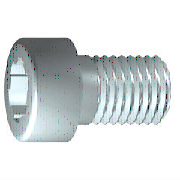
# Autodesk Inventor part: ANSI B18.3 - 4-40 UNC - 0.25, SSHCSI
Saved by Autodesk Inventor 2023.2 (Build 272271000, 271)
## iProperties
Created: 2022-02-04
Part Number: ANSI B18.3 - 4-40 UNC - 0.25, SSHCSI
Material: Steel, Mild
Description: Hexagon Socket Head Cap Screw
Document SubType Name: Modeling
Standard: ANSI B18.3
Designer: Nathan Cai
Standard Revision: 2003
Standards Organization: ANSI
Language: en-US
Size Designation: 4-40 UNC - 0.25
Categories: <MemberInstance><Categories><Category DisplayName="Fasteners" InternalName="e4da775c-781d-43d5-af7c-5136215cf5a6" Mnemonic="FSTN"><Category DisplayName="Bolts" InternalName="536e6df0-f778-49ac-b2f2-25c71d2aa0b2" Mnemonic="SCRW"><CategoryParameter DisplayName="Nominal Diameter Designation" InternalName="03caf894-eafd-4c09-a035-916ac084b87b" Mnemonic="nomdiadesig"/><CategoryParameter DisplayName="Nominal Length" InternalName="238ecbaf-3e6c-45dd-aa95-4068c8e0fd02" Mnemonic="nomlen"/><CategoryParameter DisplayName="Thread Designation" InternalName="586d5e89-370a-4089-914f-0110033585c7" Mnemonic="thrdesign"/><CategoryParameter DisplayName="Thread Series Designation" InternalName="87c5849c-b3a5-4c3e-9c9b-2feecef9be86" Mnemonic="thrserdsgn"/><CategoryParameter DisplayName="Nominal Diameter" InternalName="8bbe3f8e-44cf-40a9-a251-3a6edc8168d6" Mnemonic="nomdia"/><CategoryParameter DisplayName="Thread Type" InternalName="b4bbb7bc-d6aa-4c9f-a9a9-4152b9f6fe49" Mnemonic="thrtype"/><CategoryParameter DisplayName="Thread Pitch" InternalName="bb82302e-82d8-4176-8fc1-c5d7bb17d5ad" Mnemonic="pitch1"/><CategoryParameter DisplayName="Threads per Unit" InternalName="bdc6e7d2-ffd0-4d9c-a173-16b95ebb912d" Mnemonic="thrperunit1"/><CategoryParameter DisplayName="Thread Class" InternalName="ebc0d23b-2cc6-4d2a-b376-d52aae53bab6" Mnemonic="thrclss"/><Category DisplayName="Socket Head" InternalName="55e06bf3-7e58-486c-bbdc-745fcc60664d" Mnemonic="CLSCRW"><CategoryParameter DisplayName="Shank Diameter" InternalName="179dbae3-102f-48bb-85fe-1e3ecd34f7cc" Mnemonic="grpdia"/><CategoryParameter DisplayName="Thread Length" InternalName="3268731d-5f9a-4750-8b01-4a959c46fbf2" Mnemonic="thrlen"/><CategoryParameter DisplayName="Head Diameter" InternalName="46177176-dbdd-4a1b-aefd-4c60c45016af" Mnemonic="headdia"/><CategoryParameter DisplayName="Grip Length" InternalName="52eab69f-422f-4795-9995-175a1b827e67" Mnemonic="grplen"/><CategoryParameter DisplayName="Type" InternalName="59a7e495-7a0c-4a5c-bdfd-c090c5f6e2db" Mnemonic="type"/><CategoryParameter DisplayName="Head Height" InternalName="99c92c4c-4a02-4ebe-9e64-948fb169e19e" Mnemonic="headh"/></Category></Category></Category><Category DisplayName="DataType" InternalName="23b78d0f-2648-40c6-8793-ca6db495c9e8" Mnemonic="DATATYPE"><CategoryParameter DisplayName="DisplayName" InternalName="05415f3d-3907-474b-a020-eb9d644f4cf3" Mnemonic="DISPLAYNAME"/><CategoryParameter DisplayName="Standard" InternalName="0c0a119c-1e12-4c84-803f-101930972f5e" Mnemonic="STANDARD"/><CategoryParameter DisplayName="Description" InternalName="13903e3d-64b1-4950-80da-f627842ea37f" Mnemonic="DESCRIPTION"/><CategoryParameter DisplayName="Designation" InternalName="2675968c-4ce5-49e0-a4f5-552d29089031" Mnemonic="DESIGNATION"/><CategoryParameter DisplayName="Default Row" InternalName="2af9ec52-faaa-4026-b378-f9fa4afca842" Mnemonic="DEFAULTROW"/><CategoryParameter DisplayName="Folder Name" InternalName="3f06958e-8713-4116-9be7-ed6184ecc97b" Mnemonic="FOLDERNAME"/><CategoryParameter DisplayName="Revision Guid" InternalName="45a75005-10b1-4dfc-8d6d-dfe629f0b93c" Mnemonic="REVISIONGUID"/><CategoryParameter DisplayName="FileName" InternalName="8b46a4cc-9585-4fed-90c3-899f57e09a73" Mnemonic="FILENAME"/><CategoryParameter DisplayName="StdsOrg" InternalName="8f5914e1-4693-403f-8ab5-d37768198c9d" Mnemonic="STDSORG"/><CategoryParameter DisplayName="Family Version" InternalName="914462f6-6e19-4b14-ba84-155b9680b1d0" Mnemonic="FAMILYREVISION"/><CategoryParameter DisplayName="Standard Revision" InternalName="91d5a463-65c2-4fde-b823-3b7fea5e8e17" Mnemonic="STANDARDREVISION"/><CategoryParameter DisplayName="Member Revision" InternalName="a65d44b9-392f-4f4f-857b-e4b3d54996fe" Mnemonic="MEMBERREVISION"/><CategoryParameter DisplayName="ClipFormat" InternalName="bc51e27b-3422-4e78-93ef-cec197ddf230" Mnemonic="CLIPFORMAT"/><CategoryParameter DisplayName="Manufacturer" InternalName="cd6c7a72-a28a-4e50-99a9-2c7f4e13e5ad" Mnemonic="MANUFACTURER"/><CategoryParameter DisplayName="InternalName" InternalName="cf1d0246-76d9-4b4a-8305-fa0409afb5c1" Mnemonic="INTERNALNAME"/><CategoryParameter DisplayName="IsMetric" InternalName="e2385c5b-1ea4-4823-96a8-8de651266ec3" Mnemonic="ISMETRIC"/><Category DisplayName="Part" InternalName="c0e0b642-3bcb-4cc8-9e80-f96d35c4afa4" Mnemonic="PART"><CategoryParameter DisplayName="Part Number" InternalName="016b6077-bfbe-49bd-92c9-d8d59c39c941" Mnemonic="PARTNUMBER"/><CategoryParameter DisplayName="Stock Number" InternalName="4dba7c1c-e26c-444e-836c-b08b433409a8" Mnemonic="STOCKNUMBER"/><CategoryParameter DisplayName="Material Key" InternalName="5c9a8adb-dd2b-4535-b97f-0a94a95fe41f" Mnemonic="MATERIALKEY"/><CategoryParameter DisplayName="Material" InternalName="818a152a-d3c3-49ca-80ee-df7d91421b8e" Mnemonic="MATERIAL"/></Category></Category><Category DisplayName="Legacy Map DA" InternalName="924fff40-ddd0-4eff-ad42-30e3774ef79e" Mnemonic="LEGACYMAPDA"><CategoryParameter DisplayName="DACookie" InternalName="316934ee-8fe1-4c7a-9c36-f2d79e1add1a" Mnemonic="DACOOKIE"/></Category><Category DisplayName="LegacyMap" InternalName="cd87c42b-3e48-431e-b5c0-1cbeb14dfe77" Mnemonic="LEGACYMAP"><CategoryParameter DisplayName="unique DA member ID" InternalName="0918ad47-427f-4fed-ae26-24c81c58f590" Mnemonic="DACOOKIE"/><CategoryParameter DisplayName="Merge11 ID" InternalName="0ee8fb18-e2ed-4f39-96f6-1f4b5f50aa71" Mnemonic="MERGE11"/><CategoryParameter DisplayName="unique CC member ID" InternalName="5193edd4-b2b0-4ab4-9d54-de900eee34e0" Mnemonic="CCCOOKIE"/><CategoryParameter DisplayName="Split ID" InternalName="72b5c83c-be7f-45c4-ae51-9160ea6deb26" Mnemonic="SPLIT"/><CategoryParameter DisplayName="MemberID" InternalName="8e5e0294-fc51-4c8f-b3d7-003dc5ed94f6" Mnemonic="MEMBERID"/><CategoryParameter DisplayName="CatalogName" InternalName="d99d1e27-aa94-4de2-af4c-c348882a6f4f" Mnemonic="CATALOGNAME"/><CategoryParameter DisplayName="FamilyNumber" InternalName="e705e1f4-09cb-413e-91f9-551b4188271e" Mnemonic="FAMILYNUMBER"/></Category></Categories><FamilyTemplate Id="sis145"><FamilyTemplateParameters><FamilyTemplateParameter ObjectType="kUserParameterObject" ValueType="xs:double" Id="1" ObjectReferenceKey="GUL"/><FamilyTemplateParameter ObjectType="kUserParameterObject" ValueType="xs:double" Id="2" ObjectReferenceKey="KOH"/><FamilyTemplateParameter ObjectType="kUserParameterObject" ValueType="xs:double" Id="3" ObjectReferenceKey="NLG"/><FamilyTemplateParameter ObjectType="kUserParameterObject" ValueType="xs:double" Id="4" ObjectReferenceKey="KOD"/><FamilyTemplateParameter ObjectType="kUserParameterObject" ValueType="xs:double" Id="5" ObjectReferenceKey="SBR"/><FamilyTemplateParameter ObjectType="kUserParameterObject" ValueType="xs:double" Id="6" ObjectReferenceKey="TOA"/><FamilyTemplateParameter ObjectType="kUserParameterObject" ValueType="xs:double" Id="7" ObjectReferenceKey="GD1"/><FamilyTemplateParameter ObjectType="kUserParameterObject" ValueType="xs:double" Id="8" ObjectReferenceKey="GEL"/><FamilyTemplateParameter ObjectType="kUserParameterObject" ValueType="xs:double" Id="9" ObjectReferenceKey="SW"/><FamilyTemplateParameter ObjectType="kUserParameterObject" ValueType="xs:double" Id="10" ObjectReferenceKey="THREADDIA"/><FamilyTemplateParameter ObjectType="kUserParameterObject" ValueType="xs:double" Id="11" ObjectReferenceKey="SPD"/><FamilyTemplateParameter ObjectType="kUserParameterObject" ValueType="xs:double" Id="12" ObjectReferenceKey="INTI"/><FamilyTemplateParameter ObjectType="kUserParameterObject" ValueType="xs:double" Id="13" ObjectReferenceKey="BDM"/><FamilyTemplateParameter ObjectType="kUserParameterObject" ValueType="xs:double" Id="14" ObjectReferenceKey="ANZ"/><FamilyTemplateParameter ObjectType="kUserParameterObject" ValueType="xs:double" Id="15" ObjectReferenceKey="RR"/><FamilyTemplateParameter ObjectType="kUserParameterObject" ValueType="xs:double" Id="16" ObjectReferenceKey="TPU"/><FamilyTemplateParameter ObjectType="kUserParameterObject" ValueType="xs:double" Id="17" ObjectReferenceKey="PTC"/><FamilyTemplateParameter ObjectType="kUserParameterObject" ValueType="xs:double" Id="18" ObjectReferenceKey="NND"/><FamilyTemplateParameter ObjectType="kUserParameterObject" ValueType="xs:double" Id="19" ObjectReferenceKey="GD"/><FamilyTemplateParameter ObjectType="kUserParameterObject" ValueType="xs:double" Id="20" ObjectReferenceKey="GAL"/><FamilyTemplateParameter ObjectType="kUserParameterObject" ValueType="xs:double" Id="21" ObjectReferenceKey="E0"/><FamilyTemplateParameter ObjectType="kPropertyObject" ValueType="xs:string" Id="100" ObjectReferenceKey="{32853F0F-3444-11d1-9E93-0060B03C1CA6}" SubObjectId="52"/><FamilyTemplateParameter ObjectType="kPropertyObject" ValueType="xs:string" Id="105" ObjectReferenceKey="{32853F0F-3444-11d1-9E93-0060B03C1CA6}" SubObjectId="5"/><FamilyTemplateParameter ObjectType="kPartComponentDefinitionObject" ValueType="xs:string" Id="110" SubObjectId="Material"/><FamilyTemplateParameter ObjectType="kThreadFeatureObject" ValueType="xs:structure" Id="300" ObjectReferenceKey="100200001000000000100000000000008000000000000000" SubObjectId="ThreadInfo"><FamilyTemplateParameter ObjectType="" ValueType="xs:string" Id="301" SubObjectId="ThreadDesignation"/><FamilyTemplateParameter ObjectType="" ValueType="xs:string" Id="302" SubObjectId="ThreadType"/><FamilyTemplateParameter ObjectType="" ValueType="xs:string" Id="303" SubObjectId="ThreadClass"/></FamilyTemplateParameter></FamilyTemplateParameters></FamilyTemplate><CategoryParameterMap><ParamToTemplateMap><ParamToTemplate CategoryParameter="//CategoryParameter[@InternalName='05415f3d-3907-474b-a020-eb9d644f4cf3']" ConstantValue="Spline Socket Head Cap Screw - Inch"/><ParamToTemplate CategoryParameter="//CategoryParameter[@InternalName='cf1d0246-76d9-4b4a-8305-fa0409afb5c1']" ConstantValue="48533e16-23c5-4596-a6af-3b71bb979595"/><ParamToTemplate CategoryParameter="//CategoryParameter[@InternalName='3f06958e-8713-4116-9be7-ed6184ecc97b']" ConstantValue="ANSI B18.3(13)"/><ParamToTemplate CategoryParameter="//CategoryParameter[@InternalName='914462f6-6e19-4b14-ba84-155b9680b1d0']" ConstantValue="10"/><ParamToTemplate CategoryParameter="//CategoryParameter[@InternalName='bc51e27b-3422-4e78-93ef-cec197ddf230']" ConstantValue="CF_INVENTOR.STDPARTS"/><ParamToTemplate CategoryParameter="//CategoryParameter[@InternalName='e2385c5b-1ea4-4823-96a8-8de651266ec3']" ConstantValue="false"/><ParamToTemplate CategoryParameter="//CategoryParameter[@InternalName='13903e3d-64b1-4950-80da-f627842ea37f']" ConstantValue="Hexagon Socket Head Cap Screw"/><ParamToTemplate CategoryParameter="//CategoryParameter[@InternalName='8f5914e1-4693-403f-8ab5-d37768198c9d']" ConstantValue="ANSI"/><ParamToTemplate CategoryParameter="//CategoryParameter[@InternalName='0c0a119c-1e12-4c84-803f-101930972f5e']" ConstantValue="ANSI B18.3"/><ParamToTemplate CategoryParameter="//CategoryParameter[@InternalName='cd6c7a72-a28a-4e50-99a9-2c7f4e13e5ad']" TemplateParameter="104"/><ParamToTemplate CategoryParameter="//CategoryParameter[@InternalName='91d5a463-65c2-4fde-b823-3b7fea5e8e17']" ConstantValue="2003"/><ParamToTemplate CategoryParameter="//CategoryParameter[@InternalName='45a75005-10b1-4dfc-8d6d-dfe629f0b93c']" ConstantValue="427e49c2-ecb5-4fa3-b939-1b6f11ba86db"/><ParamToTemplate CategoryParameter="//CategoryParameter[@InternalName='2af9ec52-faaa-4026-b378-f9fa4afca842']" ConstantValue="110"/><ParamToTemplate CategoryParameter="//CategoryParameter[@InternalName='d99d1e27-aa94-4de2-af4c-c348882a6f4f']" ConstantValue="ANSI"/><ParamToTemplate CategoryParameter="//CategoryParameter[@InternalName='8b46a4cc-9585-4fed-90c3-899f57e09a73']" ConstantValue="ANSI B18.3 - 4-40 UNC - 0.25(22)"/><ParamToTemplate CategoryParameter="//CategoryParameter[@InternalName='a65d44b9-392f-4f4f-857b-e4b3d54996fe']" ConstantValue="0708E7DF-237C-4B0D-ACF9-FA1811921CFF"/><ParamToTemplate CategoryParameter="//CategoryParameter[@InternalName='52eab69f-422f-4795-9995-175a1b827e67']" ConstantValue="0.0625"/><ParamToTemplate CategoryParameter="//CategoryParameter[@InternalName='ebc0d23b-2cc6-4d2a-b376-d52aae53bab6']" ConstantValue="2A"/><ParamToTemplate CategoryParameter="//CategoryParameter[@InternalName='87c5849c-b3a5-4c3e-9c9b-2feecef9be86']" ConstantValue="UNC"/><ParamToTemplate CategoryParameter="//CategoryParameter[@InternalName='03caf894-eafd-4c09-a035-916ac084b87b']" ConstantValue="#4"/><ParamToTemplate CategoryParameter="//CategoryParameter[@InternalName='b4bbb7bc-d6aa-4c9f-a9a9-4152b9f6fe49']" ConstantValue="ANSI Unified Screw Threads"/><ParamToTemplate CategoryParameter="//CategoryParameter[@InternalName='e705e1f4-09cb-413e-91f9-551b4188271e']" ConstantValue="155"/><ParamToTemplate CategoryParameter="//CategoryParameter[@InternalName='8e5e0294-fc51-4c8f-b3d7-003dc5ed94f6']" ConstantValue="4040"/><ParamToTemplate CategoryParameter="//CategoryParameter[@InternalName='316934ee-8fe1-4c7a-9c36-f2d79e1add1a']" ConstantValue="*Ans~AB18_3_2~No. 4-40x0.25~0.25~UNRC*"/><ParamToTemplate CategoryParameter="//CategoryParameter[@InternalName='179dbae3-102f-48bb-85fe-1e3ecd34f7cc']" TemplateParameter="13"/><ParamToTemplate CategoryParameter="//CategoryParameter[@InternalName='2675968c-4ce5-49e0-a4f5-552d29089031']" TemplateParameter="100"/><ParamToTemplate CategoryParameter="//CategoryParameter[@InternalName='3268731d-5f9a-4750-8b01-4a959c46fbf2']" TemplateParameter="8"/><ParamToTemplate CategoryParameter="//CategoryParameter[@InternalName='46177176-dbdd-4a1b-aefd-4c60c45016af']" TemplateParameter="4"/><ParamToTemplate CategoryParameter="//CategoryParameter[@InternalName='99c92c4c-4a02-4ebe-9e64-948fb169e19e']" TemplateParameter="2"/><ParamToTemplate CategoryParameter="//CategoryParameter[@InternalName='818a152a-d3c3-49ca-80ee-df7d91421b8e']" TemplateParameter="110"/><ParamToTemplate CategoryParameter="//CategoryParameter[@InternalName='238ecbaf-3e6c-45dd-aa95-4068c8e0fd02']" TemplateParameter="3"/><ParamToTemplate CategoryParameter="//CategoryParameter[@InternalName='8bbe3f8e-44cf-40a9-a251-3a6edc8168d6']" TemplateParameter="18"/><ParamToTemplate CategoryParameter="//CategoryParameter[@InternalName='016b6077-bfbe-49bd-92c9-d8d59c39c941']" TemplateParameter="105"/><ParamToTemplate CategoryParameter="//CategoryParameter[@InternalName='bb82302e-82d8-4176-8fc1-c5d7bb17d5ad']" TemplateParameter="17"/><ParamToTemplate CategoryParameter="//CategoryParameter[@InternalName='586d5e89-370a-4089-914f-0110033585c7']" TemplateParameter="301"/><ParamToTemplate CategoryParameter="//CategoryParameter[@InternalName='bdc6e7d2-ffd0-4d9c-a173-16b95ebb912d']" TemplateParameter="16"/></ParamToTemplateMap></CategoryParameterMap></MemberInstance>
Density: 7.85 g/cm^3
Appearance: Semi-Polished
IsCustomPart: 0
Author: Nathan Cai
Autodesk Inventor part; units mm, degrees
ref_plane "YZ Plane" through (0, 0, 0) normal (1, 0, 0) x (0, 1, 0)
sketch "Sketch1" plane through (0, 0, 0) normal (0, 0, 1) x (1, 0, 0)
  line L0 (-2.8448, 0) -> (6.35, 0)
  line L1 (6.35, 0) -> (6.35, 1.4224)
  line L2 (6.35, 1.4224) -> (0, 1.4224)
  line L3 (0, 1.4224) -> (0, 2.3241)
  line L4 (-7.3162, 0) -> (16.036, 0) projected
  line L5 (0, -0.4648) -> (0, 2.7889) projected
  line L6 (0, 2.3241) -> (-2.8448, 2.3241)
  line L7 (-2.8448, 0) -> (-2.8448, 2.3241)
  arc A0 (-1.1734, 0) -> (-1.5494, 1.4034) centre (-3.9802, 0) ccw
  line L8 (-2.8448, 1.4034) -> (-1.5494, 1.4034)
  line L9 (12.7, 1.4224) -> (0, 1.4224) construction
  dimension "d0" = 6.35
  dimension "d1" = 2.8448
  dimension "d2" = 2.8448
  dimension "d5" = 4.6482
  dimension "d13" = 2.8068
  dimension "d14" = 2.8068
  dimension "d15" = 1.2954
  constraints: 16 end point, 5 point on line, 3 parallel, 3 perpendicular, 2 collinear, 2 point on circle, 1 centre point, 1 horizontal
  measures "d0" distance between parallel lines of L1 L3
  measures "d1" distance from line of L0.start L3
  measures "d2" diameter of L2 L0
  measures "d5" diameter of L3.end L0
  measures "d13" radius of A0
  measures "d14" diameter of L8 L0
  measures "d15" distance from line of L8.end L7
revolve "Body" add sketch "Sketch1" angle 360 about axis through (-2.8448, 0, 0) along (1, 0, 0) contours A0 L8 L7 L6 L3 L5 L0 | L5 L2 L1 L0
ref_plane "IDS_WORKPLANE{1}" through (-2.8448, 0, 0) normal (1, 0, 0) x (0, 0, -1)
sketch "Sketch2" plane through (-2.8448, 0, 0) normal (1, 0, 0) x (0, 0, -1)
  line L0 (0, -3.6027) -> (0, 5.3473) projected
  line L1 (5.6384, 0) -> (-3.6512, 0) projected
  circle A0 centre (0, 0) radius 2.3241 projected
  line L2 (1.3655, 0.3238) -> (1.1714, 0.3239)
  line L3 (0, 0) -> (1.3655, 0.3238) construction
  line L4 (0, 0) -> (4.3113, 4.0687) construction
  line L5 (0, 0) -> (0.4023, 1.3445) construction
  line L6 (0, 0) -> (0.7017, 1.2154) construction
  line L7 (0.4023, 1.3445) -> (0.3053, 1.1764)
  line L8 (0.9632, 1.0207) -> (0.8662, 0.8526)
  line L9 (0, 0) -> (0.9632, 1.0207) construction
  arc A1 (1.2154, 0) -> (1.1714, 0.3239) centre (0, 0) ccw
  arc A2 (0.8662, 0.8526) -> (0.3053, 1.1764) centre (0, 0) ccw
  arc A3 (1.4034, 0) -> (1.3655, 0.3238) centre (0, 0) ccw
  arc A4 (0.9632, 1.0207) -> (0.4023, 1.3445) centre (0, 0) ccw
  arc A5 (1.3655, 0.3238) -> (0.8276, 1.1334) centre (0, 0) ccw construction
  arc A6 (1.1714, 0.3239) -> (0.8662, 0.8526) centre (0, 0) ccw construction
  line L10 (1.3655, -0.3238) -> (1.1714, -0.3239)
  line L11 (0.4023, -1.3445) -> (0.3053, -1.1764)
  line L12 (0.9632, -1.0207) -> (0.8662, -0.8526)
  arc A7 (1.1714, -0.3239) -> (1.2154, 0) centre (0, 0) ccw
  arc A8 (0.3053, -1.1764) -> (0.8662, -0.8526) centre (0, 0) ccw
  arc A9 (1.3655, -0.3238) -> (1.4034, 0) centre (0, 0) ccw
  arc A10 (0.4023, -1.3445) -> (0.9632, -1.0207) centre (0, 0) ccw
  line L13 (-1.3655, 0.3238) -> (-1.1714, 0.3239)
  line L14 (-0.4023, 1.3445) -> (-0.3053, 1.1764)
  line L15 (-0.9632, 1.0207) -> (-0.8662, 0.8526)
  arc A11 (-1.1714, 0.3239) -> (-1.2154, 0) centre (0, 0) ccw
  arc A12 (-0.3053, 1.1764) -> (-0.8662, 0.8526) centre (0, 0) ccw
  arc A13 (-1.3655, 0.3238) -> (-1.4034, 0) centre (0, 0) ccw
  arc A14 (-0.4023, 1.3445) -> (-0.9632, 1.0207) centre (0, 0) ccw
  line L16 (-0.4023, -1.3445) -> (-0.3053, -1.1764)
  arc A15 (-0.8662, -0.8526) -> (-0.3053, -1.1764) centre (0, 0) ccw
  line L17 (-0.9632, -1.0207) -> (-0.8662, -0.8526)
  arc A16 (-0.9632, -1.0207) -> (-0.4023, -1.3445) centre (0, 0) ccw
  arc A17 (-1.2154, 0) -> (-1.1714, -0.3239) centre (0, 0) ccw
  line L18 (-1.3655, -0.3238) -> (-1.1714, -0.3239)
  arc A18 (-1.4034, 0) -> (-1.3655, -0.3238) centre (0, 0) ccw
  point P0 (0.7017, -1.2154)
  point P1 (-0.7017, 1.2154)
  point P2 (-0.7017, -1.2154)
  dimension "d19" = 0.3239
  dimension "d20" = 0.6477
  dimension "d21" = 33.316
  dimension "d22" = 2.8068
  dimension "d23" = 2.4308
  constraints: 40 point on circle, 34 end point, 26 symmetric about line, 18 centre point, 7 coincident, 2 parallel, 2 point on line, 23 other
  measures "d19" distance between parallel lines of L2 L1
  measures "d20" distance between parallel lines of L7 L8
  measures "d21" angle of L9 L3
  measures "d22" diameter of A5
  measures "d23" diameter of A6
extrude "Slot" add sketch "Sketch2" along normal up to next contours A1 L2 A3 L1 | L1 A9 L10 A7 | A17 L18 A18 L1 | L1 A13 L13 A11 | A4 L8 A2 L7 | L11 A8 L12 A10 | L14 A12 L15 A14 | A16 L17 A15 L16
fillet "Fillet1" radius 0.2286 1 edges at (-2.8448, -2.3241, 0)
thread "Thread" size "4-40 UNC" class "2A" standard "ANSI Unified Screw Threads" length 4.7625
chamfer "Chamfer1" distance 0.3785 distance2 0.3785 1 edges at (6.35, -1.4224, 0) measured on face at (6.35, -0.3549, 0.3144)
ref_plane "Work Plane2" through (-1.4224, 0, 0) normal (0, 0, -1) x (1, 0, 0)
equation "\"d19\" = 0.5 * SBR"
equation "\"d20\" = SBR"
equation "\"d22\" = 1.1547 * SW"
equation "\"d23\" = SW"
equation "\"d17\" = INTI"
equation "\"d24\" = RR"
equation "\"d6\" = GEL"
equation "\"d9\" = -0.5 * SPD + 0.5 * NND"
equation "\"d10\" = GUL"
equation "\"d0\" = NLG"
equation "\"d1\" = KOH"
equation "\"d2\" = NND"
equation "\"d5\" = KOD"
equation "\"d13\" = 1.1547 * SW"
equation "\"d14\" = 1.1547 * SW"
equation "\"d15\" = INTI"
equation "\"NND\" = 2.8448"
equation "\"NLG\" = 6.35"
equation "\"GEL\" = 4.7625"
equation "\"KOD\" = 4.6482"
equation "\"KOH\" = 2.8448"
equation "\"SPD\" = GD1"
equation "\"GUL\" = 0.37846"
equation "\"SBR\" = 0.6477"
equation "\"INTI\" = 1.2954"
equation "\"d11\" = -KOH"
equation "\"SW\" = 2.43078"
equation "\"d16\" = 1.1547 * SW"
equation "\"d18\" = SW"
equation "\"RR\" = 0.2286"
equation "\"TOA\" = 30deg"
equation "\"GD1\" = 2.08788"
equation "\"THREADDIA\" = 2.8448"
equation "\"BDM\" = NND"
equation "\"GD\" = NND"
equation "\"GAL\" = 1.5875"
equation "\"E0\" = 2.86258"
body "Solid1"
